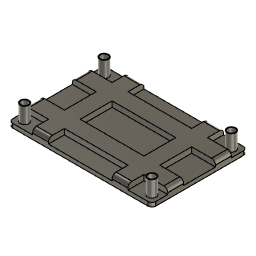
force_plate (Autodesk Fusion 360 design; units mm, degrees)
Autodesk Fusion 360 part; units mm, degrees
note: some values were not read from the file. Chosen so that the rebuilt part matches the saved one: which face or edge a step refers to.
sketch "Sketch1" plane through (0, 0, 0) normal (0, 0, 1) x (1, 0, 0)
  line L0 (90, -60) -> (-90, -60)
  line L1 (-90, -60) -> (-90, 60)
  line L2 (-90, 60) -> (90, 60)
  line L3 (90, 60) -> (90, -60)
  line L4 (90, -60) -> (-90, 60) construction
  line L5 (-90, -60) -> (90, 60) construction
  circle A0 centre (-80, 50) radius 5
  circle A1 centre (-80, -50) radius 5
  circle A2 centre (80, 50) radius 5
  circle A3 centre (80, -50) radius 5
  dimension "d1" = 180
  dimension "d2" = 120
  dimension "d3" = 10
  dimension "d4" = 10
  dimension "d5" = 10
  dimension "d6" = 10
  constraint horizontal L0
  constraint perpendicular L0 L1
  constraint parallel L0 L2
  constraint parallel L1 L3
  constraint coincident L4 origin
  constraint coincident L5 origin
  measures "d1" distance of L1.end L2.end
  measures "d2" distance of L0.end L1.end
  measures "d3" diameter of A0
  measures "d4" diameter of A1
  measures "d5" diameter of A2
  measures "d6" diameter of A3
extrude "Extrude1" add sketch "Sketch1" along normal blind 5 makes body 1
move_face "MoveFace1" by (0, -115, 0) 1 faces at (-25.2896, 15.7278, 5) on bodies 1
move_body "Move1" bodies 1 to x (1, 0, 0) y (0, 1, 0) z (0, 0, 1) at (0, -200, 0)
sketch "Sketch2" plane through (0, 0, 0) normal (0, 0, 1) x (1, 0, 0)
  line L0 (90, -60) -> (-90, -60)
  line L1 (-90, -60) -> (-90, 60)
  line L2 (-90, 60) -> (90, 60)
  line L3 (90, 60) -> (90, -60)
  line L4 (90, -60) -> (-90, 60) construction
  line L5 (-90, -60) -> (90, 60) construction
  dimension "d9" = 180
  dimension "d10" = 120
  constraint horizontal L0
  constraint perpendicular L0 L1
  constraint parallel L0 L2
  constraint parallel L1 L3
  constraint coincident L4 origin
  constraint coincident L5 origin
  measures "d9" distance of L1.end L2.end
  measures "d10" distance of L0.end L1.end
sketch "Sketch3" plane through (0, 0, 5) normal (0, 0, 1) x (-1, 0, 0)
  line L0 (-90, -60) -> (90, -60)
  line L1 (90, -60) -> (90, 60)
  line L2 (90, 60) -> (-90, 60)
  line L3 (-90, 60) -> (-90, -60)
sketch "Sketch4" plane through (0, 0, 5) normal (0, 0, 1) x (-1, 0, 0)
  circle A0 centre (-80, 50) radius 4
  circle A1 centre (80, 50) radius 4
  circle A2 centre (-80, -50) radius 4
  circle A3 centre (80, -50) radius 4
  dimension "d13" = 8
  dimension "d14" = 8
  dimension "d15" = 8
  dimension "d16" = 8
  measures "d13" diameter of A0
  measures "d14" diameter of A1
  measures "d15" diameter of A2
  measures "d16" diameter of A3
sketch "Sketch5" plane through (0, 0, 5) normal (0, 0, 1) x (-1, 0, 0)
  line L0 (22.5, -15) -> (-22.5, -15)
  line L1 (-22.5, -15) -> (-22.5, 15)
  line L2 (-22.5, 15) -> (22.5, 15)
  line L3 (22.5, 15) -> (22.5, -15)
  line L4 (22.5, -15) -> (-22.5, 15) construction
  line L5 (-22.5, -15) -> (22.5, 15) construction
  dimension "d19" = 45
  dimension "d20" = 30
  constraint horizontal L0
  constraint perpendicular L0 L1
  constraint parallel L0 L2
  constraint parallel L1 L3
  constraint coincident L4 origin
  constraint coincident L5 origin
  measures "d19" distance of L1.end L2.end
  measures "d20" distance of L0.end L1.end
sketch "Sketch6" plane through (0, 0, 15) normal (0, 0, 1) x (-1, 0, 0)
  line L0 (22.5, 15) -> (-22.5, 15)
  line L1 (-22.5, 15) -> (-22.5, -15)
  line L2 (-22.5, -15) -> (22.5, -15)
  line L3 (22.5, -15) -> (22.5, 15)
  circle A0 centre (17, 0) radius 1
  circle A1 centre (-17, 0) radius 1
  dimension "d23" = 17
  dimension "d24" = 17
  dimension "d25" = 2
  dimension "d26" = 2
  measures "d23" distance of origin A1.centre
  measures "d24" distance of origin A0.centre
  measures "d25" diameter of A0
  measures "d26" diameter of A1
extrude "Extrude5" cut sketch "Sketch6" against normal blind 9 contours A0 | A1
extrude "Extrude6" cut 4 faces at (-25.2896, -184.2722, 0) (-25.2896, -184.2722, 0) (-25.2896, -184.2722, 0) (-25.2896, -184.2722, 0) along direction (0, 0, -1) blind 10 on bodies 1
extrude "Extrude7" cut 1 faces at (-25.2896, -184.2722, 0) along direction (0, 0, -1) blind 10 on bodies 1 makes body 2
sketch "Sketch7" plane through (0, 0, 2) normal (0, 0, 1) x (-1, 0, 0)
  circle A0 centre (-80, -50) radius 4
  circle A1 centre (80, 50) radius 4
  circle A2 centre (-80, 50) radius 4
  circle A3 centre (80, -50) radius 4
  line L0 (-90, 60) -> (-90, -60)
  line L1 (-90, -60) -> (90, -60)
  line L2 (90, -60) -> (90, 60)
  line L3 (90, 60) -> (-90, 60)
  line L4 (22.5, 15) -> (-22.5, 15)
  line L5 (-22.5, 15) -> (-22.5, -15)
  line L6 (-22.5, -15) -> (22.5, -15)
  line L7 (22.5, -15) -> (22.5, 15)
  line L8 (22.5, 15) -> (-22.5, -15) construction
  line L9 (-22.5, 15) -> (22.5, -15) construction
  dimension "d39" = 45
  dimension "d40" = 30
  constraint horizontal L4
  constraint perpendicular L4 L5
  constraint parallel L4 L6
  constraint parallel L5 L7
  constraint coincident L8 origin
  constraint coincident L9 origin
  measures "d39" distance of L5.end L6.end
  measures "d40" distance of L4.end L5.end
sketch "Sketch8" plane through (0, 0, 8) normal (0, 0, 1) x (-1, 0, 0)
  line L0 (22.5, -15) -> (22.5, 15)
  line L1 (22.5, 15) -> (-22.5, 15)
  line L2 (-22.5, 15) -> (-22.5, -15)
  line L3 (-22.5, -15) -> (22.5, -15)
  circle A0 centre (-17, 0) radius 1
  circle A1 centre (17, 0) radius 1
  dimension "d43" = 17
  dimension "d44" = 17
  dimension "d45" = 2
  dimension "d46" = 2
  measures "d43" distance of origin A1.centre
  measures "d44" distance of origin A0.centre
  measures "d45" diameter of A0
  measures "d46" diameter of A1
extrude "Extrude15" cut 1 faces at (-25.2896, -184.2722, 5) along direction (0, 0, -1) blind 3 on bodies 1 bodies 1
sketch "Sketch9" plane through (0, 0, 2) normal (0, 0, 1) x (-1, 0, 0)
  circle A0 centre (80, 150) radius 5
  circle A1 centre (-80, 150) radius 5
  circle A2 centre (80, 250) radius 5
  circle A3 centre (-80, 250) radius 5
  line L0 (-90, 140) -> (90, 140)
  line L1 (90, 140) -> (90, 260)
  line L2 (90, 260) -> (-90, 260)
  line L3 (-90, 260) -> (-90, 140)
extrude "Extrude16" add sketch "Sketch9" against normal blind 2 contours A0 | A1 | A2 | A3 bodies 1
sketch "Sketch10" plane through (0, 0, 2) normal (0, 0, 1) x (-1, 0, 0)
  line L0 (-90, 140) -> (90, 140)
  line L1 (90, 140) -> (90, 260)
  line L2 (90, 260) -> (-90, 260)
  line L3 (-90, 260) -> (-90, 140)
  circle A0 centre (80, 150) radius 4.5
  circle A1 centre (-80, 150) radius 4.5
  circle A2 centre (80, 250) radius 4.5
  circle A3 centre (-80, 250) radius 4.5
  circle A4 centre (80, 250) radius 5.5
  circle A5 centre (80, 150) radius 5.5
  circle A6 centre (-80, 150) radius 5.5
  circle A7 centre (-80, 250) radius 5.5
  dimension "d59" = 9
  dimension "d60" = 9
  dimension "d61" = 9
  dimension "d62" = 9
  dimension "d63" = 11
  dimension "d64" = 11
  dimension "d65" = 11
  dimension "d66" = 11
  constraint concentric A2 A4
  constraint concentric A0 A5
  constraint concentric A1 A6
  constraint concentric A3 A7
  measures "d59" diameter of A0
  measures "d60" diameter of A1
  measures "d61" diameter of A2
  measures "d62" diameter of A3
  measures "d63" diameter of A4
  measures "d64" diameter of A5
  measures "d65" diameter of A6
  measures "d66" diameter of A7
extrude "Extrude17" add sketch "Sketch10" along normal blind 10 contours A4 | A5 | A6 | A7 bodies 1
fillet "Fillet2" radius 5 4 edges at (90, -260, 1) (-90, -260, 1) (-90, -140, 1) (90, -140, 1) on bodies 1
extrude "Extrude18" add 4 faces at (-75.2449, -148.0133, 12) (-84.7551, -248.0133, 12) (75.0019, -248.7442, 12) (77.1903, -154.3201, 12) along direction (0, 0, 1) blind 10 on bodies 1 bodies 1
sketch "Sketch11" plane through (0, 0, 2) normal (0, 0, 1) x (-1, 0, 0)
  circle A0 centre (80, 150) radius 5.5
  circle A1 centre (80, 250) radius 5.5
  arc A2 (-90, 145) -> (-85, 140) centre (-85, 145) ccw
  line L0 (-85, 140) -> (85, 140)
  arc A3 (85, 140) -> (90, 145) centre (85, 145) ccw
  line L1 (90, 145) -> (90, 255)
  arc A4 (90, 255) -> (85, 260) centre (85, 255) ccw
  line L2 (85, 260) -> (-85, 260)
  arc A5 (-85, 260) -> (-90, 255) centre (-85, 255) ccw
  line L3 (-90, 255) -> (-90, 145)
  circle A6 centre (-80, 250) radius 5.5
  circle A7 centre (-80, 150) radius 5.5
  line L4 (-22.5, 215) -> (22.5, 215)
  line L5 (22.5, 215) -> (22.5, 185)
  line L6 (22.5, 185) -> (-22.5, 185)
  line L7 (-22.5, 185) -> (-22.5, 215)
  line L8 (-22.5, 215) -> (22.5, 185) construction
  line L9 (22.5, 215) -> (-22.5, 185) construction
  line L10 (60, 140) -> (40, 140)
  line L11 (40, 140) -> (40, 260)
  line L12 (40, 260) -> (60, 260)
  line L13 (60, 260) -> (60, 140)
  line L14 (-40, 140) -> (-60, 140)
  line L15 (-60, 140) -> (-60, 260)
  line L16 (-60, 260) -> (-40, 260)
  line L17 (-40, 260) -> (-40, 140)
  line L18 (90, 160) -> (-90, 160)
  line L19 (-90, 160) -> (-90, 180)
  line L20 (-90, 180) -> (90, 180)
  line L21 (90, 180) -> (90, 160)
  line L22 (90, 220) -> (-90, 220)
  line L23 (-90, 220) -> (-90, 240)
  line L24 (-90, 240) -> (90, 240)
  line L25 (90, 240) -> (90, 220)
  point P0 (0, 200)
  dimension "d73" = 45
  dimension "d74" = 30
  constraint horizontal L4
  constraint perpendicular L4 L5
  constraint parallel L4 L6
  constraint parallel L5 L7
  constraint coincident L8 P0
  constraint coincident L9 P0
  constraint horizontal L10
  constraint vertical L11
  constraint horizontal L12
  constraint vertical L13
  constraint coincident L2 L11.end
  constraint coincident L0 L10.start
  constraint horizontal L14
  constraint vertical L15
  constraint horizontal L16
  constraint vertical L17
  constraint coincident L2 L15.end
  constraint coincident L0 L14.start
  constraint horizontal L18
  constraint vertical L19
  constraint horizontal L20
  constraint vertical L21
  constraint coincident L3 L19.end
  constraint horizontal L22
  constraint vertical L23
  constraint horizontal L24
  constraint vertical L25
  constraint coincident L3 L23.end
  constraint coincident L1 L22.start
  measures "d73" distance of L5.end L6.end
  measures "d74" distance of L4.end L5.end
extrude "Extrude19" add sketch "Sketch11" along normal blind 7 contours L3 L15 L18 L19 L20 | L0 L14 L15 L17 L18 | L15 L17 L18 L20 | L3 L15 L22 L23 L24 | L15 L17 L20 L22 | L11 L17 L18 L20 | L0 L10 L11 L13 L18 | L15 L17 L22 L24 | L11 L13 L18 L20 | L2 L15 L16 L17 L24 | L11 L17 L22 L24 | L11 L13 L20 L22 | L1 L13 L18 L20 L21 | L11 L13 L22 L24 | L2 L11 L12 L13 L24 | L1 L13 L22 L24 L25 bodies 1
fillet "Fillet3" radius 5 8 edges at (-50, -260, 9) (50, -260, 9) (90, -230, 9) (90, -170, 9) (50, -140, 9) (-50, -140, 9) (-90, -170, 9) (-90, -230, 9) on bodies 1
extrude "Extrude20" add 1 faces at (28.3333, -220, 0) along direction (0, 0, -1) blind 3 on bodies 1 bodies 1
sketch "Sketch12" plane through (0, 0, 0) normal (1, 0, 0) x (0, 1, 0)
named bodies: "plate"
